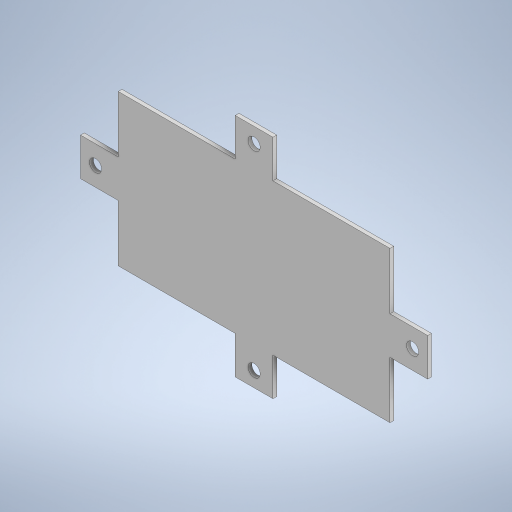
# Autodesk Inventor part: base
Saved by Autodesk Inventor 2023 (Build 270158000, 158)
## iProperties
Created: 2023-05-28
Part Number: base
Material: 一般
Document SubType Name: Sheet Metal
Designer: 310611102
Density: 1 g/cm^3
Sheet Metal Rule: Default_mm
Appearance: 預設
Author: 310611102
Autodesk Inventor part; units mm, degrees
ref_plane "YZ Plane" through (0, 0, 0) normal (1, 0, 0) x (0, 1, 0)
ref_plane "XZ Plane" through (0, 0, 0) normal (0, 1, 0) x (-1, 0, 0)
ref_plane "XY Plane" through (0, 0, 0) normal (0, 0, 1) x (1, 0, 0)
sketch "Sketch1" plane through (0, 0, 0) normal (0, 0, 1) x (1, 0, 0)
  line L0 (-36, 20) -> (36, 20)
  line L1 (36, 20) -> (36, -20)
  line L2 (36, -20) -> (-36, -20)
  line L3 (-36, -20) -> (-36, 20)
  line L4 (-36, 20) -> (36, -20) construction
  line L5 (36, 20) -> (-36, -20) construction
  point P0 (0, 0)
  dimension "d0" = 40
  dimension "d1" = 72
  measures "d0" distance of L0.end L1.end
  measures "d1" distance of L0.start L0.end
sketch "Sketch2" plane through (0, 0, 1) normal (0, 0, 1) x (1, 0, 0)
  line L0 (-36, 20) -> (36, 20)
  line L1 (-46, -5) -> (-36, -5)
  line L2 (-36, -5) -> (-36, 5)
  line L3 (-36, 5) -> (-46, 5)
  line L4 (-46, 5) -> (-46, -5)
  line L5 (-46, -5) -> (-36, 5) construction
  line L6 (-36, -5) -> (-46, 5) construction
  line L7 (0, 0) -> (0, 7.0571)
  line L8 (0, 0) -> (6.6312, 0)
  line L9 (-36, -20) -> (-36, 20)
  line L10 (46, -5) -> (36, -5)
  line L11 (36, -5) -> (36, 5)
  line L12 (36, 5) -> (46, 5)
  line L13 (46, 5) -> (46, -5)
  line L14 (46, -5) -> (36, 5) construction
  line L15 (36, -5) -> (46, 5) construction
  circle A0 centre (-42, 0) radius 1.6
  circle A1 centre (42, 0) radius 1.6
  line L16 (36, -20) -> (-36, -20)
  line L17 (-5, -30) -> (5, -30)
  line L18 (5, -30) -> (5, -20)
  line L19 (5, -20) -> (-5, -20)
  line L20 (-5, -20) -> (-5, -30)
  line L21 (-5, -30) -> (5, -20) construction
  line L22 (5, -30) -> (-5, -20) construction
  circle A2 centre (0, -26) radius 1.6
  line L23 (-5, 30) -> (5, 30)
  line L24 (5, 30) -> (5, 20)
  line L25 (5, 20) -> (-5, 20)
  line L26 (-5, 20) -> (-5, 30)
  line L27 (-5, 30) -> (5, 20) construction
  line L28 (5, 30) -> (-5, 20) construction
  circle A3 centre (0, 26) radius 1.6
  point P0 (-41, 0)
  point P1 (41, 0)
  point P2 (0, -25)
  point P3 (0, 25)
  dimension "d5" = 10
  dimension "d6" = 10
  dimension "d10" = 3.2
  dimension "d12" = 4
  dimension "d18" = 3.2
  dimension "d19" = 10
  dimension "d20" = 10
  dimension "d21" = 4
  measures "d5" distance of L2.end L3.end
  measures "d6" distance of L3.end L1.start
  measures "d10" diameter of A0
  measures "d12" distance from line of L4 A0.centre
  measures "d18" diameter of A2
  measures "d19" distance of L17.start L17.end
  measures "d20" distance of L19.end L17.start
  measures "d21" distance from line of L17 A2.centre
sketch "Sketch3" plane through (0, 0, 1) normal (0, 0, 1) x (1, 0, 0)
  line L0 (-22.5, 27.5) -> (-12.5, 27.5)
  line L1 (-7.5, 22.5) -> (-7.5, 12.5)
  line L2 (-12.5, 7.5) -> (-22.5, 7.5)
  line L3 (-27.5, 12.5) -> (-27.5, 22.5)
  line L4 (-27.5, 27.5) -> (-7.5, 7.5) construction
  line L5 (-7.5, 27.5) -> (-27.5, 7.5) construction
  line L6 (-11.1923, 0) -> (11.1923, 0)
  line L7 (0, 8.4231) -> (0, -8.4231)
  arc A0 (-22.5, 27.5) -> (-27.5, 22.5) centre (-22.5, 22.5) ccw
  arc A1 (-7.5, 22.5) -> (-12.5, 27.5) centre (-12.5, 22.5) ccw
  arc A2 (-12.5, 7.5) -> (-7.5, 12.5) centre (-12.5, 12.5) ccw
  arc A3 (-27.5, 12.5) -> (-22.5, 7.5) centre (-22.5, 12.5) ccw
  line L8 (22.5, 27.5) -> (12.5, 27.5)
  line L9 (7.5, 22.5) -> (7.5, 12.5)
  line L10 (12.5, 7.5) -> (22.5, 7.5)
  line L11 (27.5, 12.5) -> (27.5, 22.5)
  line L12 (27.5, 27.5) -> (7.5, 7.5) construction
  line L13 (7.5, 27.5) -> (27.5, 7.5) construction
  arc A4 (27.5, 22.5) -> (22.5, 27.5) centre (22.5, 22.5) ccw
  arc A5 (12.5, 27.5) -> (7.5, 22.5) centre (12.5, 22.5) ccw
  arc A6 (7.5, 12.5) -> (12.5, 7.5) centre (12.5, 12.5) ccw
  arc A7 (22.5, 7.5) -> (27.5, 12.5) centre (22.5, 12.5) ccw
  line L14 (-22.5, -27.5) -> (-12.5, -27.5)
  line L15 (-7.5, -22.5) -> (-7.5, -12.5)
  line L16 (-12.5, -7.5) -> (-22.5, -7.5)
  line L17 (-27.5, -12.5) -> (-27.5, -22.5)
  line L18 (-27.5, -27.5) -> (-7.5, -7.5) construction
  line L19 (-7.5, -27.5) -> (-27.5, -7.5) construction
  arc A8 (-27.5, -22.5) -> (-22.5, -27.5) centre (-22.5, -22.5) ccw
  arc A9 (-12.5, -27.5) -> (-7.5, -22.5) centre (-12.5, -22.5) ccw
  arc A10 (-7.5, -12.5) -> (-12.5, -7.5) centre (-12.5, -12.5) ccw
  arc A11 (-22.5, -7.5) -> (-27.5, -12.5) centre (-22.5, -12.5) ccw
  line L20 (7.5, -22.5) -> (7.5, -12.5)
  arc A12 (12.5, -7.5) -> (7.5, -12.5) centre (12.5, -12.5) ccw
  arc A13 (7.5, -22.5) -> (12.5, -27.5) centre (12.5, -22.5) ccw
  line L21 (22.5, -27.5) -> (12.5, -27.5)
  line L22 (12.5, -7.5) -> (22.5, -7.5)
  line L23 (27.5, -27.5) -> (7.5, -7.5) construction
  line L24 (7.5, -27.5) -> (27.5, -7.5) construction
  arc A14 (27.5, -12.5) -> (22.5, -7.5) centre (22.5, -12.5) ccw
  line L25 (27.5, -12.5) -> (27.5, -22.5)
  arc A15 (22.5, -27.5) -> (27.5, -22.5) centre (22.5, -22.5) ccw
  point P0 (0, 0)
  point P1 (-17.5, 17.5)
  point P2 (0, 0)
  point P3 (17.5, 17.5)
  point P4 (-17.5, -17.5)
  point P5 (17.5, -17.5)
  dimension "d29" = 20
  dimension "d30" = 15
  dimension "d31" = 15
  dimension "d32" = 20
  dimension "d33" = 5
  constraints: 52 end point, 51 symmetric about line, 32 point on circle, 32 point on line, 16 centre point, 8 tangent, 4 midpoint, 3 equal radius, 2 horizontal, 2 parallel, 1 coincident, 1 perpendicular, 1 vertical, 12 other
  measures "d29" distance between parallel lines of L2 L0
  measures "d30" diameter of L1 L7
  measures "d31" diameter of L2 L6
  measures "d32" distance of L4.start L5.start
  measures "d33" radius of A0
extrude "Plate1" add sketch "Sketch1" along normal blind 1
sheet face with bend "Face2" sketch "Sketch2" thickness 1 toward (0, 0, -1) bend radius 1 relief straight relief width 1 relief depth 0.5
bend "Bend1"
equation "\"d2\" = 厚度"
equation "\"d13\" = 折彎半徑"
equation "\"d14\" = 折彎離隙寬度"
equation "\"d16\" = 最小剩餘"
equation "\"d15\" = 折彎離隙深度"
equation "\"d17\" = 轉移半徑"
equation "\"折彎半徑\" = 厚度"
equation "\"折彎離隙寬度\" = 厚度"
equation "\"折彎離隙深度\" = 0.5 * 厚度"
equation "\"轉角離隙大小\" = 4 * 厚度"
equation "\"最小剩餘\" = 2 * 厚度"
equation "\"轉移半徑\" = 折彎半徑"
equation "\"Jacobi半徑大小\" = 折彎半徑"
equation "\"間隙大小\" = 厚度"
equation "\"厚度\" = 1"
body "Solid1"
